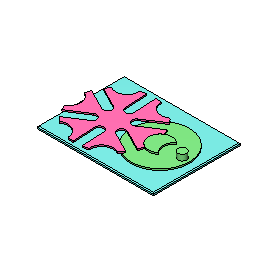
Homework 4 v1 (Autodesk Fusion 360 design; units mm, degrees)
Autodesk Fusion 360 part; units mm, degrees
sketch "Holder" plane through (0, 0, 0) normal (0, 0, 1) x (1, 0, 0) in component "Holder"
  line L0 (200, 150) -> (-200, 150)
  line L1 (-200, 150) -> (-200, -150)
  line L2 (-200, -150) -> (200, -150)
  line L3 (200, -150) -> (200, 150)
  line L4 (200, 150) -> (-200, -150) construction
  line L5 (-200, 150) -> (200, -150) construction
  dimension "d1" = 400
  dimension "d2" = 300
  constraint horizontal L0
  constraint perpendicular L0 L1
  constraint parallel L0 L2
  constraint parallel L1 L3
  constraint coincident L4 origin
  constraint coincident L5 origin
  measures "d1" distance of L1.end L2.end
  measures "d2" distance of L0.end L1.end
extrude "Extrude1" add sketch "Holder" along normal blind 8 makes body 1 in component "Holder"
chamfer "Chamfer1" distance 3 angle 45 1 edges at (0, -150, 8) on bodies 1 in component "Holder"
chamfer "Chamfer1" distance 3 angle 45 3 edges at (200, 0, 8) (0, 150, 8) (-200, 0, 8) on bodies 1 in component "Holder"
sketch "Crank" plane through (0, 0, 8) normal (0, 0, 1) x (-1, 0, 0) in component "Crank"
  line L0 (-197, -147) -> (197, -147)
  line L1 (197, -147) -> (197, 147)
  line L2 (197, 147) -> (-197, 147)
  line L3 (-197, 147) -> (-197, -147)
  circle A0 centre (-73.5, 0) radius 100
  dimension "d7" = 200
  measures "d7" diameter of A0
extrude "Extrude1'" add sketch "Crank" along normal blind 5 separate body contours A0 makes body 2 in component "Crank"
sketch "Crank-holder" plane through (0, 0, 8) normal (0, 0, -1) x (1, 0, 0) in component "Crank"
  circle A0 centre (73.5, 0) radius 100
  circle A1 centre (73.5, 0) radius 10
  dimension "d10" = 20
  constraint concentric A0 A1
  measures "d10" diameter of A1
extrude "Extrude2" add sketch "Crank-holder" along normal blind 8 contours A1 bodies 2 in component "Crank"
extrude "Extrude2'" cut sketch "Crank-holder" along normal blind 50 contours A1 bodies 1 in component "Holder"
move_face "OffsetFaces1" offset -0.3 1 faces at (83.4503, -0.9957, 2.6667) on bodies 1 in component "Holder"
sketch "Crank moon pin" plane through (0, 0, 13) normal (0, 0, 1) x (-1, 0, 0) in component "Crank"
  circle A0 centre (-73.5, 0) radius 100
  arc A1 (-99.0265, -30.7961) -> (-99.0265, 30.7961) centre (-73.5, 0) ccw
  arc A2 (-99.0265, -30.7961) -> (-99.0265, 30.7961) centre (-124.553, 0) ccw
  dimension "d16" = 80
  dimension "d17" = 80
  constraint concentric A0 A1
  measures "d16" diameter of A1
  measures "d17" diameter of A2
sketch "Crank pin" plane through (0, 0, 13) normal (0, 0, 1) x (-1, 0, 0) in component "Crank"
  circle A0 centre (-148.6727, -0.766) radius 15
  dimension "d18" = 30
  measures "d18" diameter of A0
extrude "Extrude3" add sketch "Crank moon pin" along normal blind 5 contours A1 A2 bodies 2 in component "Crank"
extrude "Extrude4" add sketch "Crank pin" along normal blind 20 bodies 2 in component "Crank"
sketch "Flower" plane through (0, 0, 13) normal (0, 0, 1) x (-1, 0, 0) in component "Flower"
  circle A0 centre (-148.6727, -0.766) radius 15
  arc A1 (-99.0265, -30.7961) -> (-99.0265, 30.7961) centre (-124.553, 0) ccw
  arc A2 (-99.0265, -30.7961) -> (-99.0265, 30.7961) centre (-73.5, 0) ccw
  circle A3 centre (-73.5, 0) radius 100
  arc A4 (-52.7381, -34.1898) -> (-56.5183, 36.2163) centre (-73.5, 0) ccw
  arc A5 (47.9184, -124.1524) -> (-14.9452, -92.2231) centre (7.9282, -125.0378) ccw
  arc A6 (176.1565, -81.9626) -> (117.0731, -120.4394) centre (156.9282, -117.0378) ccw
  arc A7 (203.7381, 50.1898) -> (207.5183, -20.2163) centre (224.5, 16) ccw
  arc A8 (103.0816, 140.1524) -> (165.9452, 108.2231) centre (143.0718, 141.0378) ccw
  arc A9 (-25.1565, 97.9626) -> (33.9269, 136.4394) centre (-5.9282, 133.0378) ccw
  line L0 (-33.8417, -63.2064) -> (-19.9889, -84.4782)
  line L1 (-25.656, -75.776) -> (37.5972, -34.5838)
  line L2 (-42.0274, -50.6369) -> (21.2258, -9.4446)
  line L3 (-25.656, -75.776) -> (-28.7402, -77.7845)
  line L4 (-42.0274, -50.6369) -> (-45.1115, -52.6454)
  arc A10 (-52.7381, -34.1898) -> (-45.1115, -52.6454) centre (75.5, 8) ccw
  arc A11 (-28.7402, -77.7845) -> (-14.9452, -92.2231) centre (75.5, 8) ccw
  arc A12 (37.5972, -34.5838) -> (21.2258, -9.4446) centre (29.4115, -22.0142) ccw
  line L5 (97.4742, -121.4917) -> (97.6715, -125.1669)
  line L6 (97.4742, -121.4917) -> (93.4272, -46.1167)
  line L7 (67.5173, -123.1001) -> (67.7147, -126.7753)
  line L8 (67.5173, -123.1001) -> (63.4703, -47.7251)
  arc A13 (93.4272, -46.1167) -> (63.4703, -47.7251) centre (78.4488, -46.9209) ccw
  line L9 (198.6302, -37.7156) -> (201.9117, -39.3824)
  line L10 (198.6302, -37.7156) -> (131.33, -3.5329)
  line L11 (185.0447, -64.4632) -> (188.3262, -66.13)
  line L12 (185.0447, -64.4632) -> (117.7445, -30.2805)
  arc A14 (131.33, -3.5329) -> (117.7445, -30.2805) centre (124.5373, -16.9067) ccw
  line L13 (176.656, 91.776) -> (179.7402, 93.7845)
  line L14 (176.656, 91.776) -> (113.4028, 50.5838)
  line L15 (193.0274, 66.6369) -> (196.1115, 68.6454)
  line L16 (193.0274, 66.6369) -> (129.7742, 25.4446)
  arc A15 (113.4028, 50.5838) -> (129.7742, 25.4446) centre (121.5885, 38.0142) ccw
  line L17 (53.5258, 137.4917) -> (53.3285, 141.1669)
  line L18 (53.5258, 137.4917) -> (57.5728, 62.1167)
  line L19 (83.4827, 139.1001) -> (83.2853, 142.7753)
  line L20 (83.4827, 139.1001) -> (87.5297, 63.7251)
  arc A16 (57.5728, 62.1167) -> (87.5297, 63.7251) centre (72.5512, 62.9209) ccw
  line L21 (-47.6302, 53.7156) -> (-50.9117, 55.3824)
  line L22 (-47.6302, 53.7156) -> (19.67, 19.5329)
  line L23 (-34.0447, 80.4632) -> (-37.3262, 82.13)
  line L24 (-34.0447, 80.4632) -> (33.2555, 46.2805)
  arc A17 (19.67, 19.5329) -> (33.2555, 46.2805) centre (26.4627, 32.9067) ccw
  arc A18 (47.9184, -124.1524) -> (67.7147, -126.7753) centre (75.5, 8) ccw
  arc A19 (97.6715, -125.1669) -> (117.0731, -120.4394) centre (75.5, 8) ccw
  arc A20 (176.1565, -81.9626) -> (188.3262, -66.13) centre (75.5, 8) ccw
  arc A21 (201.9117, -39.3824) -> (207.5183, -20.2163) centre (75.5, 8) ccw
  arc A22 (203.7381, 50.1898) -> (196.1115, 68.6454) centre (75.5, 8) ccw
  arc A23 (179.7402, 93.7845) -> (165.9452, 108.2231) centre (75.5, 8) ccw
  arc A24 (103.0816, 140.1524) -> (83.2853, 142.7753) centre (75.5, 8) ccw
  arc A25 (53.3285, 141.1669) -> (33.9269, 136.4394) centre (75.5, 8) ccw
  arc A26 (-25.1565, 97.9626) -> (-37.3262, 82.13) centre (75.5, 8) ccw
  arc A27 (-50.9117, 55.3824) -> (-56.5183, 36.2163) centre (75.5, 8) ccw
  dimension "d33" = 270
  dimension "d34" = 80
  dimension "d36" = 360
  dimension "d39" = 30
  dimension "d40" = 15
  dimension "d41" = 15
  dimension "d43" = 360
  constraint coincident A2 A4.end
  constraint coincident A2 A4.start
  constraint concentric A2 A4
  constraint concentric A10 A18
  constraint concentric A18 A20
  constraint concentric A20 A22
  constraint concentric A22 A24
  constraint concentric A24 A26
  constraint tangent L1 A12
  constraint tangent L2 A12
  constraint coincident L3.end A10
  constraint coincident A3 L0.end
  constraint concentric A10 A11
  constraint concentric A18 A19
  constraint concentric A20 A21
  constraint concentric A22 A23
  constraint concentric A24 A25
  constraint concentric A26 A27
  measures "d33" diameter of A10
  measures "d34" diameter of A4
  measures "d39" diameter of A12
  measures "d40" distance of L0.start L1.start
  measures "d41" distance of L0.start L2.start
extrude "Extrude1''" add sketch "Flower" along normal blind 5 separate body contours A2 A3 A4 L2 L4 A10 A12 L21 L22 A17 A27 | A3 A5 A6 A7 A8 A9 L1 A11 A12 L5 L6 L7 L8 A13 L9 L10 L11 L12 A14 L13 L14 L15 L16 A15 L17 L18 L19 L20 A16 L24 A17 A18 A19 A20 A21 A22 A23 A24 A25 A26 | A3 L0 L1 | A3 L23 L24 A26 | A3 L0 L3 A11 makes body 3 in component "Flower"
move_face "OffsetFaces1'" offset -0.1 1 faces at (133.6914, 1.5137, 26.3333) on bodies 2 in component "Crank"
sketch "Flower-holder" plane through (0, 0, 13) normal (0, 0, -1) x (1, 0, 0) in component "Flower"
  line L0 (50.9117, 55.3824) -> (-19.67, 19.5329)
  arc A0 (-33.2555, 46.2805) -> (-19.67, 19.5329) centre (-26.4627, 32.9067) ccw
  line L1 (-33.2555, 46.2805) -> (37.3262, 82.13)
  arc A1 (37.3262, 82.13) -> (25.1565, 97.9626) centre (-75.5, 8) ccw
  arc A2 (-33.9269, 136.4394) -> (25.1565, 97.9626) centre (5.9282, 133.0378) ccw
  arc A3 (-33.9269, 136.4394) -> (-53.3285, 141.1669) centre (-75.5, 8) ccw
  line L2 (-53.3285, 141.1669) -> (-57.5728, 62.1167)
  arc A4 (-87.5297, 63.7251) -> (-57.5728, 62.1167) centre (-72.5512, 62.9209) ccw
  line L3 (-87.5297, 63.7251) -> (-83.2853, 142.7753)
  arc A5 (-83.2853, 142.7753) -> (-103.0816, 140.1524) centre (-75.5, 8) ccw
  arc A6 (-165.9452, 108.2231) -> (-103.0816, 140.1524) centre (-143.0718, 141.0378) ccw
  arc A7 (-165.9452, 108.2231) -> (-179.7402, 93.7845) centre (-75.5, 8) ccw
  line L4 (-179.7402, 93.7845) -> (-113.4028, 50.5838)
  arc A8 (-129.7742, 25.4446) -> (-113.4028, 50.5838) centre (-121.5885, 38.0142) ccw
  line L5 (-129.7742, 25.4446) -> (-196.1115, 68.6454)
  arc A9 (-196.1115, 68.6454) -> (-203.7381, 50.1898) centre (-75.5, 8) ccw
  arc A10 (-207.5183, -20.2163) -> (-203.7381, 50.1898) centre (-224.5, 16) ccw
  arc A11 (-207.5183, -20.2163) -> (-201.9117, -39.3824) centre (-75.5, 8) ccw
  line L6 (-201.9117, -39.3824) -> (-131.33, -3.5329)
  arc A12 (-117.7445, -30.2805) -> (-131.33, -3.5329) centre (-124.5373, -16.9067) ccw
  line L7 (-117.7445, -30.2805) -> (-188.3262, -66.13)
  arc A13 (-188.3262, -66.13) -> (-176.1565, -81.9626) centre (-75.5, 8) ccw
  arc A14 (-117.0731, -120.4394) -> (-176.1565, -81.9626) centre (-156.9282, -117.0378) ccw
  arc A15 (-117.0731, -120.4394) -> (-97.6715, -125.1669) centre (-75.5, 8) ccw
  line L8 (-97.6715, -125.1669) -> (-93.4272, -46.1167)
  arc A16 (-63.4703, -47.7251) -> (-93.4272, -46.1167) centre (-78.4488, -46.9209) ccw
  line L9 (-63.4703, -47.7251) -> (-67.7147, -126.7753)
  arc A17 (-67.7147, -126.7753) -> (-47.9184, -124.1524) centre (-75.5, 8) ccw
  arc A18 (14.9452, -92.2231) -> (-47.9184, -124.1524) centre (-7.9282, -125.0378) ccw
  arc A19 (14.9452, -92.2231) -> (28.7402, -77.7845) centre (-75.5, 8) ccw
  line L10 (28.7402, -77.7845) -> (-37.5972, -34.5838)
  arc A20 (-21.2258, -9.4446) -> (-37.5972, -34.5838) centre (-29.4115, -22.0142) ccw
  line L11 (-21.2258, -9.4446) -> (45.1115, -52.6454)
  arc A21 (45.1115, -52.6454) -> (52.7381, -34.1898) centre (-75.5, 8) ccw
  arc A22 (56.5183, 36.2163) -> (52.7381, -34.1898) centre (73.5, 0) ccw
  arc A23 (56.5183, 36.2163) -> (50.9117, 55.3824) centre (-75.5, 8) ccw
  circle A24 centre (-75.5, 8) radius 15
  dimension "d47" = 30
  constraint concentric A1 A24
  measures "d47" diameter of A24
extrude "Extrude2''" add sketch "Flower-holder" along normal blind 13 contours A24 bodies 3 in component "Flower"
extrude "Extrude3'" cut sketch "Flower-holder" along normal blind 40 contours A24 bodies 1 in component "Holder"
move_face "OffsetFaces2" offset -0.3 1 faces at (-60.5186, -8.7477, 5.3333) on bodies 1 in component "Holder"
move_face "OffsetFaces2'" offset -0.3 1 faces at (97.4982, -32.0014, 16.3333) on bodies 2 in component "Crank"
component "Holder" placed x (1, 0, 0) y (0, 1, 0) z (0, 0, 1) at (0, 0, 0)
component "Crank" placed x (1, 0, 0) y (0, 1, 0) z (0, 0, 1) at (0, 0, 0)
component "Flower" placed x (1, 0, 0) y (0, 1, 0) z (0, 0, 1) at (0, 0, 0)
named bodies: "Holder", "Crank", "Flower"
